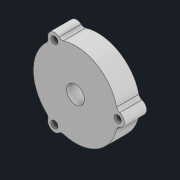
# Autodesk Inventor part: Motor Spacer
Saved by Autodesk Inventor 2021 (Build 250183000, 183)
## iProperties
Created: 2020-10-18
Part Number: Motor Spacer
Material: Generic
Document SubType Name: Modeling
Designer: Eugene Tang
Mass: 172.726 g
Surface Area: 253.223 cm^2
Volume: 172.726 cm^3
Density: 1 g/cm^3
Appearance: Default
Author: Eugene Tang
Autodesk Inventor part; units mm, degrees
ref_plane "YZ Plane" through (0, 0, 0) normal (1, 0, 0) x (0, 1, 0)
ref_plane "XZ Plane" through (0, 0, 0) normal (0, 1, 0) x (-1, 0, 0)
sketch "Sketch1" plane through (0, 0, 0) normal (0, 0, 1) x (1, 0, 0)
  circle A0 centre (0, -10) radius 10 projected
  circle A1 centre (47.5, -10) radius 4 projected
  arc A2 (-13.75, -55.4663) -> (46.25, -20.8253) centre (0, -10) ccw projected
  arc A3 (49.6711, -17.1789) -> (46.25, -20.8253) centre (51.1184, -21.9648) ccw projected
  arc A4 (49.6711, -17.1789) -> (49.6711, -2.8211) centre (47.5, -10) ccw projected
  arc A5 (46.25, 0.8253) -> (49.6711, -2.8211) centre (51.1184, 1.9648) ccw projected
  arc A6 (46.25, 0.8253) -> (-13.75, 35.4663) centre (0, -10) ccw projected
  arc A7 (-18.6184, 36.6058) -> (-13.75, 35.4663) centre (-15.1974, 40.2523) ccw projected
  arc A8 (-18.6184, 36.6058) -> (-31.0526, 29.4269) centre (-23.75, 31.1362) ccw projected
  arc A9 (-32.5, 24.641) -> (-31.0526, 29.4269) centre (-35.9211, 28.2874) ccw projected
  arc A10 (-32.5, 24.641) -> (-47.4342, -7.5) centre (0, -10) ccw projected
  line L0 (-47.5, -7.5) -> (-47.4342, -7.5) projected
  line L1 (-47.5, -7.5) -> (-47.5, -12.5) projected
  line L2 (-47.4342, -12.5) -> (-47.5, -12.5) projected
  arc A11 (-47.4342, -12.5) -> (-32.5, -44.641) centre (0, -10) ccw projected
  arc A12 (-31.0526, -49.4269) -> (-32.5, -44.641) centre (-35.9211, -48.2874) ccw projected
  arc A13 (-31.0526, -49.4269) -> (-18.6184, -56.6058) centre (-23.75, -51.1362) ccw projected
  arc A14 (-13.75, -55.4663) -> (-18.6184, -56.6058) centre (-15.1974, -60.2523) ccw projected
  circle A15 centre (-23.75, 31.1362) radius 4 projected
  circle A16 centre (-23.75, -51.1362) radius 4 projected
  point P0 (0, 0)
  constraints: 1 vertical alignment
ref_plane "Work Plane1" through (-44.1783, -54.1783, 25) normal (0, 0, -1) x (0.3122, 0.95, 0)
extrude "Extrusion1" add sketch "Sketch1" along normal up to surface (25 mm away)
body "Solid1"
